Autodesk Inventor part; units mm, degrees
(part 3 of 4)
sketch "Sketch6" plane through (0, 0, 2) normal (0, 0, 1) x (1, 0, 0)
  line L0 (283.7872, -294.4284) -> (283.7872, -329.9768) projected
  line L1 (283.7872, -329.9768) -> (273.4247, -329.9768) projected
  line L2 (273.4247, -329.9768) -> (267.105, -323.7035) projected
  line L3 (267.105, -323.7035) -> (267.105, -286.25) projected
  line L4 (267.105, -286.25) -> (273.4247, -279.9768) projected
  line L5 (273.4247, -279.9768) -> (299.54, -279.9768) projected
  line L6 (299.54, -279.9768) -> (299.54, -294.4284) projected
  line L7 (299.54, -294.4284) -> (283.7872, -294.4284) projected
  line L8 (242.9879, -315.1998) -> (242.9879, -330.0232) projected
  line L9 (242.9879, -330.0232) -> (227.2351, -330.0232) projected
  line L10 (227.2351, -330.0232) -> (210.553, -313.3411) projected
  line L11 (210.553, -313.3411) -> (210.553, -279.9768) projected
  line L12 (210.553, -279.9768) -> (227.2351, -279.9768) projected
  line L13 (227.2351, -279.9768) -> (227.2351, -315.1998) projected
  line L14 (227.2351, -315.1998) -> (242.9879, -315.1998) projected
  line L15 (206.2779, -316.1756) -> (206.2779, -329.9768) projected
  line L16 (206.2779, -329.9768) -> (173.8429, -329.9768) projected
  line L17 (173.8429, -329.9768) -> (173.8429, -316.1756) projected
  line L18 (173.8429, -316.1756) -> (206.2779, -316.1756) projected
  line L19 (170.3113, -279.9768) -> (170.3113, -329.9768) projected
  line L20 (170.3113, -329.9768) -> (159.9954, -329.9768) projected
  line L21 (159.9954, -329.9768) -> (153.7221, -323.7035) projected
  line L22 (153.7221, -323.7035) -> (153.7221, -286.25) projected
  line L23 (153.7221, -286.25) -> (159.9954, -279.9768) projected
  line L24 (159.9954, -279.9768) -> (170.3113, -279.9768) projected
  line L25 (129.3262, -316.1292) -> (129.3262, -329.9303) projected
  line L26 (129.3262, -329.9303) -> (104.7444, -329.9303) projected
  line L27 (104.7444, -329.9303) -> (96.8913, -322.0771) projected
  line L28 (96.8913, -322.0771) -> (96.8913, -294.289) projected
  line L29 (96.8913, -294.289) -> (113.5734, -294.289) projected
  line L30 (113.5734, -294.289) -> (113.5734, -316.1292) projected
  line L31 (113.5734, -316.1292) -> (129.3262, -316.1292) projected
  line L32 (56.789, -329.9768) -> (46.6125, -329.9768) projected
  line L33 (46.6125, -329.9768) -> (40.3392, -323.7035) projected
  line L34 (40.3392, -323.7035) -> (40.3392, -279.9768) projected
  line L35 (40.3392, -279.9768) -> (56.789, -279.9768) projected
  line L36 (56.789, -279.9768) -> (56.789, -329.9768) projected
  line L37 (92.5697, -329.9768) -> (60.3206, -329.9768) projected
  line L38 (60.3206, -329.9768) -> (60.3206, -316.1756) projected
  line L39 (60.3206, -316.1756) -> (92.5697, -316.1756) projected
  line L40 (92.5697, -316.1756) -> (92.5697, -329.9768) projected
  line L41 (149.447, -294.289) -> (149.447, -329.9303) projected
  line L42 (149.447, -329.9303) -> (132.7649, -329.9303) projected
  line L43 (132.7649, -329.9303) -> (132.7649, -294.289) projected
  line L44 (132.7649, -294.289) -> (149.447, -294.289) projected
  line L45 (206.2779, -279.9768) -> (206.2779, -294.4284) projected
  line L46 (206.2779, -294.4284) -> (173.8429, -294.4284) projected
  line L47 (173.8429, -294.4284) -> (173.8429, -279.9768) projected
  line L48 (173.8429, -279.9768) -> (206.2779, -279.9768) projected
  line L49 (206.2779, -297.96) -> (206.2779, -308.973) projected
  line L50 (206.2779, -308.973) -> (173.8429, -308.973) projected
  line L51 (173.8429, -308.973) -> (173.8429, -297.96) projected
  line L52 (173.8429, -297.96) -> (206.2779, -297.96) projected
  line L53 (262.8299, -313.3411) -> (246.4266, -329.9768) projected
  line L54 (246.4266, -329.9768) -> (246.4266, -279.9768) projected
  line L55 (246.4266, -279.9768) -> (262.8299, -279.9768) projected
  line L56 (262.8299, -279.9768) -> (262.8299, -313.3411) projected
  line L57 (319.6608, -286.25) -> (319.6608, -323.7035) projected
  line L58 (319.6608, -323.7035) -> (313.3411, -329.9768) projected
  line L59 (313.3411, -329.9768) -> (287.1794, -329.9768) projected
  line L60 (287.1794, -329.9768) -> (287.1794, -316.1756) projected
  line L61 (287.1794, -316.1756) -> (302.9786, -316.1756) projected
  line L62 (302.9786, -316.1756) -> (302.9786, -279.9768) projected
  line L63 (302.9786, -279.9768) -> (313.3411, -279.9768) projected
  line L64 (313.3411, -279.9768) -> (319.6608, -286.25) projected
  line L65 (31.2247, -413) -> (28.338, -408) projected
  line L66 (28.338, -408) -> (31.2247, -403) projected
  line L67 (31.2247, -403) -> (36.9983, -403) projected
  line L68 (36.9983, -403) -> (39.885, -408) projected
  line L69 (39.885, -408) -> (36.9983, -413) projected
  line L70 (36.9983, -413) -> (31.2247, -413) projected
  line L71 (49.9886, -440.5) -> (52.8754, -445.5) projected
  line L72 (52.8754, -445.5) -> (49.9886, -450.5) projected
  line L73 (49.9886, -450.5) -> (44.2151, -450.5) projected
  line L74 (44.2151, -450.5) -> (41.3284, -445.5) projected
  line L75 (41.3284, -445.5) -> (44.2151, -440.5) projected
  line L76 (44.2151, -440.5) -> (49.9886, -440.5) projected
  line L77 (57.2247, -418) -> (62.9983, -418) projected
  line L78 (62.9983, -418) -> (65.885, -423) projected
  line L79 (65.885, -423) -> (62.9983, -428) projected
  line L80 (62.9983, -428) -> (57.2247, -428) projected
  line L81 (57.2247, -428) -> (54.338, -423) projected
  line L82 (54.338, -423) -> (57.2247, -418) projected
  line L83 (78.8754, -430.5) -> (75.9886, -435.5) projected
  line L84 (75.9886, -435.5) -> (70.2151, -435.5) projected
  line L85 (70.2151, -435.5) -> (67.3284, -430.5) projected
  line L86 (67.3284, -430.5) -> (70.2151, -425.5) projected
  line L87 (70.2151, -425.5) -> (75.9886, -425.5) projected
  line L88 (75.9886, -425.5) -> (78.8754, -430.5) projected
  line L89 (80.338, -438) -> (83.2247, -433) projected
  line L90 (83.2247, -433) -> (88.9983, -433) projected
  line L91 (88.9983, -433) -> (91.885, -438) projected
  line L92 (91.885, -438) -> (88.9983, -443) projected
  line L93 (88.9983, -443) -> (83.2247, -443) projected
  line L94 (83.2247, -443) -> (80.338, -438) projected
  line L95 (101.9886, -410.5) -> (104.8754, -415.5) projected
  line L96 (104.8754, -415.5) -> (101.9886, -420.5) projected
  line L97 (101.9886, -420.5) -> (96.2151, -420.5) projected
  line L98 (96.2151, -420.5) -> (93.3284, -415.5) projected
  line L99 (93.3284, -415.5) -> (96.2151, -410.5) projected
  line L100 (96.2151, -410.5) -> (101.9886, -410.5) projected
  line L101 (109.2247, -448) -> (114.9983, -448) projected
  line L102 (114.9983, -448) -> (117.885, -453) projected
  line L103 (117.885, -453) -> (114.9983, -458) projected
  line L104 (114.9983, -458) -> (109.2247, -458) projected
  line L105 (109.2247, -458) -> (106.338, -453) projected
  line L106 (106.338, -453) -> (109.2247, -448) projected
  line L107 (135.2247, -413) -> (132.338, -408) projected
  line L108 (132.338, -408) -> (135.2247, -403) projected
  line L109 (135.2247, -403) -> (140.9983, -403) projected
  line L110 (140.9983, -403) -> (143.885, -408) projected
  line L111 (143.885, -408) -> (140.9983, -413) projected
  line L112 (140.9983, -413) -> (135.2247, -413) projected
  line L113 (153.9886, -440.5) -> (156.8754, -445.5) projected
  line L114 (156.8754, -445.5) -> (153.9886, -450.5) projected
  line L115 (153.9886, -450.5) -> (148.2151, -450.5) projected
  line L116 (148.2151, -450.5) -> (145.3284, -445.5) projected
  line L117 (145.3284, -445.5) -> (148.2151, -440.5) projected
  line L118 (148.2151, -440.5) -> (153.9886, -440.5) projected
  line L119 (153.9886, -410.5) -> (156.8754, -415.5) projected
  line L120 (156.8754, -415.5) -> (153.9886, -420.5) projected
  line L121 (153.9886, -420.5) -> (148.2151, -420.5) projected
  line L122 (148.2151, -420.5) -> (145.3284, -415.5) projected
  line L123 (145.3284, -415.5) -> (148.2151, -410.5) projected
  line L124 (148.2151, -410.5) -> (153.9886, -410.5) projected
  line L125 (182.8754, -430.5) -> (179.9886, -435.5) projected
  line L126 (179.9886, -435.5) -> (174.2151, -435.5) projected
  line L127 (174.2151, -435.5) -> (171.3284, -430.5) projected
  line L128 (171.3284, -430.5) -> (174.2151, -425.5) projected
  line L129 (174.2151, -425.5) -> (179.9886, -425.5) projected
  line L130 (179.9886, -425.5) -> (182.8754, -430.5) projected
  line L131 (184.338, -438) -> (187.2247, -433) projected
  line L132 (187.2247, -433) -> (192.9983, -433) projected
  line L133 (192.9983, -433) -> (195.885, -438) projected
  line L134 (195.885, -438) -> (192.9983, -443) projected
  line L135 (192.9983, -443) -> (187.2247, -443) projected
  line L136 (187.2247, -443) -> (184.338, -438) projected
  line L137 (205.9886, -410.5) -> (208.8754, -415.5) projected
  line L138 (208.8754, -415.5) -> (205.9886, -420.5) projected
  line L139 (205.9886, -420.5) -> (200.2151, -420.5) projected
  line L140 (200.2151, -420.5) -> (197.3284, -415.5) projected
  line L141 (197.3284, -415.5) -> (200.2151, -410.5) projected
  line L142 (200.2151, -410.5) -> (205.9886, -410.5) projected
  line L143 (213.2247, -448) -> (218.9983, -448) projected
  line L144 (218.9983, -448) -> (221.885, -453) projected
  line L145 (221.885, -453) -> (218.9983, -458) projected
  line L146 (218.9983, -458) -> (213.2247, -458) projected
  line L147 (213.2247, -458) -> (210.338, -453) projected
  line L148 (210.338, -453) -> (213.2247, -448) projected
  line L149 (239.2247, -413) -> (236.338, -408) projected
  line L150 (236.338, -408) -> (239.2247, -403) projected
  line L151 (239.2247, -403) -> (244.9983, -403) projected
  line L152 (244.9983, -403) -> (247.885, -408) projected
  line L153 (247.885, -408) -> (244.9983, -413) projected
  line L154 (244.9983, -413) -> (239.2247, -413) projected
  line L155 (257.9886, -440.5) -> (260.8754, -445.5) projected
  line L156 (260.8754, -445.5) -> (257.9886, -450.5) projected
  line L157 (257.9886, -450.5) -> (252.2151, -450.5) projected
  line L158 (252.2151, -450.5) -> (249.3284, -445.5) projected
  line L159 (249.3284, -445.5) -> (252.2151, -440.5) projected
  line L160 (252.2151, -440.5) -> (257.9886, -440.5) projected
  line L161 (265.2247, -418) -> (270.9983, -418) projected
  line L162 (270.9983, -418) -> (273.885, -423) projected
  line L163 (273.885, -423) -> (270.9983, -428) projected
  line L164 (270.9983, -428) -> (265.2247, -428) projected
  line L165 (265.2247, -428) -> (262.338, -423) projected
  line L166 (262.338, -423) -> (265.2247, -418) projected
  line L167 (291.2247, -448) -> (296.9983, -448) projected
  line L168 (296.9983, -448) -> (299.885, -453) projected
  line L169 (299.885, -453) -> (296.9983, -458) projected
  line L170 (296.9983, -458) -> (291.2247, -458) projected
  line L171 (291.2247, -458) -> (288.338, -453) projected
  line L172 (288.338, -453) -> (291.2247, -448) projected
  line L173 (343.2247, -448) -> (348.9983, -448) projected
  line L174 (348.9983, -448) -> (351.885, -453) projected
  line L175 (351.885, -453) -> (348.9983, -458) projected
  line L176 (348.9983, -458) -> (343.2247, -458) projected
  line L177 (343.2247, -458) -> (340.338, -453) projected
  line L178 (340.338, -453) -> (343.2247, -448) projected
  line L179 (335.9886, -410.5) -> (338.8754, -415.5) projected
  line L180 (338.8754, -415.5) -> (335.9886, -420.5) projected
  line L181 (335.9886, -420.5) -> (330.2151, -420.5) projected
  line L182 (330.2151, -420.5) -> (327.3284, -415.5) projected
  line L183 (327.3284, -415.5) -> (330.2151, -410.5) projected
  line L184 (330.2151, -410.5) -> (335.9886, -410.5) projected
  line L185 (286.8754, -430.5) -> (283.9886, -435.5) projected
  line L186 (283.9886, -435.5) -> (278.2151, -435.5) projected
  line L187 (278.2151, -435.5) -> (275.3284, -430.5) projected
  line L188 (275.3284, -430.5) -> (278.2151, -425.5) projected
  line L189 (278.2151, -425.5) -> (283.9886, -425.5) projected
  line L190 (283.9886, -425.5) -> (286.8754, -430.5) projected
  line L191 (309.9886, -410.5) -> (312.8754, -415.5) projected
  line L192 (312.8754, -415.5) -> (309.9886, -420.5) projected
  line L193 (309.9886, -420.5) -> (304.2151, -420.5) projected
  line L194 (304.2151, -420.5) -> (301.3284, -415.5) projected
  line L195 (301.3284, -415.5) -> (304.2151, -410.5) projected
  line L196 (304.2151, -410.5) -> (309.9886, -410.5) projected
  line L197 (5.2247, -433) -> (10.9983, -433) projected
  line L198 (10.9983, -433) -> (13.885, -438) projected
  line L199 (13.885, -438) -> (10.9983, -443) projected
  line L200 (10.9983, -443) -> (5.2247, -443) projected
  line L201 (5.2247, -443) -> (2.338, -438) projected
  line L202 (2.338, -438) -> (5.2247, -433) projected
  line L203 (23.9886, -440.5) -> (26.8754, -445.5) projected
  line L204 (26.8754, -445.5) -> (23.9886, -450.5) projected
  line L205 (23.9886, -450.5) -> (18.2151, -450.5) projected
  line L206 (18.2151, -450.5) -> (15.3284, -445.5) projected
  line L207 (15.3284, -445.5) -> (18.2151, -440.5) projected
  line L208 (18.2151, -440.5) -> (23.9886, -440.5) projected
  line L209 (10.9983, -428) -> (5.2247, -428) projected
  line L210 (5.2247, -428) -> (2.338, -423) projected
  line L211 (2.338, -423) -> (5.2247, -418) projected
  line L212 (5.2247, -418) -> (10.9983, -418) projected
  line L213 (10.9983, -418) -> (13.885, -423) projected
  line L214 (13.885, -423) -> (10.9983, -428) projected
  line L215 (317.2247, -418) -> (322.9983, -418) projected
  line L216 (322.9983, -418) -> (325.885, -423) projected
  line L217 (325.885, -423) -> (322.9983, -428) projected
  line L218 (322.9983, -428) -> (317.2247, -428) projected
  line L219 (317.2247, -428) -> (314.338, -423) projected
  line L220 (314.338, -423) -> (317.2247, -418) projected
  line L221 (291.2247, -418) -> (296.9983, -418) projected
  line L222 (296.9983, -418) -> (299.885, -423) projected
  line L223 (299.885, -423) -> (296.9983, -428) projected
  line L224 (296.9983, -428) -> (291.2247, -428) projected
  line L225 (291.2247, -428) -> (288.338, -423) projected
  line L226 (288.338, -423) -> (291.2247, -418) projected
  line L227 (317.2247, -413) -> (314.338, -408) projected
  line L228 (314.338, -408) -> (317.2247, -403) projected
  line L229 (317.2247, -403) -> (322.9983, -403) projected
  line L230 (322.9983, -403) -> (325.885, -408) projected
  line L231 (325.885, -408) -> (322.9983, -413) projected
  line L232 (322.9983, -413) -> (317.2247, -413) projected
  line L233 (340.338, -438) -> (343.2247, -433) projected
  line L234 (343.2247, -433) -> (348.9983, -433) projected
  line L235 (348.9983, -433) -> (351.885, -438) projected
  line L236 (351.885, -438) -> (348.9983, -443) projected
  line L237 (348.9983, -443) -> (343.2247, -443) projected
  line L238 (343.2247, -443) -> (340.338, -438) projected
  line L239 (309.9886, -440.5) -> (312.8754, -445.5) projected
  line L240 (312.8754, -445.5) -> (309.9886, -450.5) projected
  line L241 (309.9886, -450.5) -> (304.2151, -450.5) projected
  line L242 (304.2151, -450.5) -> (301.3284, -445.5) projected
  line L243 (301.3284, -445.5) -> (304.2151, -440.5) projected
  line L244 (304.2151, -440.5) -> (309.9886, -440.5) projected
  line L245 (262.338, -438) -> (265.2247, -433) projected
  line L246 (265.2247, -433) -> (270.9983, -433) projected
  line L247 (270.9983, -433) -> (273.885, -438) projected
  line L248 (273.885, -438) -> (270.9983, -443) projected
  line L249 (270.9983, -443) -> (265.2247, -443) projected
  line L250 (265.2247, -443) -> (262.338, -438) projected
  line L251 (260.8754, -430.5) -> (257.9886, -435.5) projected
  line L252 (257.9886, -435.5) -> (252.2151, -435.5) projected
  line L253 (252.2151, -435.5) -> (249.3284, -430.5) projected
  line L254 (249.3284, -430.5) -> (252.2151, -425.5) projected
  line L255 (252.2151, -425.5) -> (257.9886, -425.5) projected
  line L256 (257.9886, -425.5) -> (260.8754, -430.5) projected
  line L257 (239.2247, -418) -> (244.9983, -418) projected
  line L258 (244.9983, -418) -> (247.885, -423) projected
  line L259 (247.885, -423) -> (244.9983, -428) projected
  line L260 (244.9983, -428) -> (239.2247, -428) projected
  line L261 (239.2247, -428) -> (236.338, -423) projected
  line L262 (236.338, -423) -> (239.2247, -418) projected
  line L263 (231.9886, -440.5) -> (234.8754, -445.5) projected
  line L264 (234.8754, -445.5) -> (231.9886, -450.5) projected
  line L265 (231.9886, -450.5) -> (226.2151, -450.5) projected
  line L266 (226.2151, -450.5) -> (223.3284, -445.5) projected
  line L267 (223.3284, -445.5) -> (226.2151, -440.5) projected
  line L268 (226.2151, -440.5) -> (231.9886, -440.5) projected
  line L269 (213.2247, -413) -> (210.338, -408) projected
  line L270 (210.338, -408) -> (213.2247, -403) projected
  line L271 (213.2247, -403) -> (218.9983, -403) projected
  line L272 (218.9983, -403) -> (221.885, -408) projected
  line L273 (221.885, -408) -> (218.9983, -413) projected
  line L274 (218.9983, -413) -> (213.2247, -413) projected
  line L275 (187.2247, -448) -> (192.9983, -448) projected
  line L276 (192.9983, -448) -> (195.885, -453) projected
  line L277 (195.885, -453) -> (192.9983, -458) projected
  line L278 (192.9983, -458) -> (187.2247, -458) projected
  line L279 (187.2247, -458) -> (184.338, -453) projected
  line L280 (184.338, -453) -> (187.2247, -448) projected
  line L281 (179.9886, -410.5) -> (182.8754, -415.5) projected
  line L282 (182.8754, -415.5) -> (179.9886, -420.5) projected
  line L283 (179.9886, -420.5) -> (174.2151, -420.5) projected
  line L284 (174.2151, -420.5) -> (171.3284, -415.5) projected
  line L285 (171.3284, -415.5) -> (174.2151, -410.5) projected
  line L286 (174.2151, -410.5) -> (179.9886, -410.5) projected
  line L287 (161.2247, -413) -> (158.338, -408) projected
  line L288 (158.338, -408) -> (161.2247, -403) projected
  line L289 (161.2247, -403) -> (166.9983, -403) projected
  line L290 (166.9983, -403) -> (169.885, -408) projected
  line L291 (169.885, -408) -> (166.9983, -413) projected
  line L292 (166.9983, -413) -> (161.2247, -413) projected
  line L293 (161.2247, -448) -> (166.9983, -448) projected
  line L294 (166.9983, -448) -> (169.885, -453) projected
  line L295 (169.885, -453) -> (166.9983, -458) projected
  line L296 (166.9983, -458) -> (161.2247, -458) projected
  line L297 (161.2247, -458) -> (158.338, -453) projected
  line L298 (158.338, -453) -> (161.2247, -448) projected
  line L299 (135.2247, -418) -> (140.9983, -418) projected
  line L300 (140.9983, -418) -> (143.885, -423) projected
  line L301 (143.885, -423) -> (140.9983, -428) projected
  line L302 (140.9983, -428) -> (135.2247, -428) projected
  line L303 (135.2247, -428) -> (132.338, -423) projected
  line L304 (132.338, -423) -> (135.2247, -418) projected
  line L305 (127.9886, -440.5) -> (130.8754, -445.5) projected
  line L306 (130.8754, -445.5) -> (127.9886, -450.5) projected
  line L307 (127.9886, -450.5) -> (122.2151, -450.5) projected
  line L308 (122.2151, -450.5) -> (119.3284, -445.5) projected
  line L309 (119.3284, -445.5) -> (122.2151, -440.5) projected
  line L310 (122.2151, -440.5) -> (127.9886, -440.5) projected
  line L311 (109.2247, -413) -> (106.338, -408) projected
  line L312 (106.338, -408) -> (109.2247, -403) projected
  line L313 (109.2247, -403) -> (114.9983, -403) projected
  line L314 (114.9983, -403) -> (117.885, -408) projected
  line L315 (117.885, -408) -> (114.9983, -413) projected
  line L316 (114.9983, -413) -> (109.2247, -413) projected
  line L317 (83.2247, -448) -> (88.9983, -448) projected
  line L318 (88.9983, -448) -> (91.885, -453) projected
  line L319 (91.885, -453) -> (88.9983, -458) projected
  line L320 (88.9983, -458) -> (83.2247, -458) projected
  line L321 (83.2247, -458) -> (80.338, -453) projected
  line L322 (80.338, -453) -> (83.2247, -448) projected
  line L323 (75.9886, -410.5) -> (78.8754, -415.5) projected
  line L324 (78.8754, -415.5) -> (75.9886, -420.5) projected
  line L325 (75.9886, -420.5) -> (70.2151, -420.5) projected
  line L326 (70.2151, -420.5) -> (67.3284, -415.5) projected
  line L327 (67.3284, -415.5) -> (70.2151, -410.5) projected
  line L328 (70.2151, -410.5) -> (75.9886, -410.5) projected
  line L329 (54.338, -438) -> (57.2247, -433) projected
  line L330 (57.2247, -433) -> (62.9983, -433) projected
  line L331 (62.9983, -433) -> (65.885, -438) projected
  line L332 (65.885, -438) -> (62.9983, -443) projected
  line L333 (62.9983, -443) -> (57.2247, -443) projected
  line L334 (57.2247, -443) -> (54.338, -438) projected
  line L335 (52.8754, -430.5) -> (49.9886, -435.5) projected
  line L336 (49.9886, -435.5) -> (44.2151, -435.5) projected
  line L337 (44.2151, -435.5) -> (41.3284, -430.5) projected
  line L338 (41.3284, -430.5) -> (44.2151, -425.5) projected
  line L339 (44.2151, -425.5) -> (49.9886, -425.5) projected
  line L340 (49.9886, -425.5) -> (52.8754, -430.5) projected
  line L341 (31.2247, -418) -> (36.9983, -418) projected
  line L342 (36.9983, -418) -> (39.885, -423) projected
  line L343 (39.885, -423) -> (36.9983, -428) projected
  line L344 (36.9983, -428) -> (31.2247, -428) projected
  line L345 (31.2247, -428) -> (28.338, -423) projected
  line L346 (28.338, -423) -> (31.2247, -418) projected
  line L347 (23.9886, -420.5) -> (18.2151, -420.5) projected
  line L348 (18.2151, -420.5) -> (15.3284, -415.5) projected
  line L349 (15.3284, -415.5) -> (18.2151, -410.5) projected
  line L350 (18.2151, -410.5) -> (23.9886, -410.5) projected
  line L351 (23.9886, -410.5) -> (26.8754, -415.5) projected
  line L352 (26.8754, -415.5) -> (23.9886, -420.5) projected
  line L353 (31.2247, -448) -> (36.9983, -448) projected
  line L354 (36.9983, -448) -> (39.885, -453) projected
  line L355 (39.885, -453) -> (36.9983, -458) projected
  line L356 (36.9983, -458) -> (31.2247, -458) projected
  line L357 (31.2247, -458) -> (28.338, -453) projected
  line L358 (28.338, -453) -> (31.2247, -448) projected
  line L359 (57.2247, -413) -> (54.338, -408) projected
  line L360 (54.338, -408) -> (57.2247, -403) projected
  line L361 (57.2247, -403) -> (62.9983, -403) projected
  line L362 (62.9983, -403) -> (65.885, -408) projected
  line L363 (65.885, -408) -> (62.9983, -413) projected
  line L364 (62.9983, -413) -> (57.2247, -413) projected
  line L365 (75.9886, -440.5) -> (78.8754, -445.5) projected
  line L366 (78.8754, -445.5) -> (75.9886, -450.5) projected
  line L367 (75.9886, -450.5) -> (70.2151, -450.5) projected
  line L368 (70.2151, -450.5) -> (67.3284, -445.5) projected
  line L369 (67.3284, -445.5) -> (70.2151, -440.5) projected
  line L370 (70.2151, -440.5) -> (75.9886, -440.5) projected
  line L371 (83.2247, -418) -> (88.9983, -418) projected
  line L372 (88.9983, -418) -> (91.885, -423) projected
  line L373 (91.885, -423) -> (88.9983, -428) projected
  line L374 (88.9983, -428) -> (83.2247, -428) projected
  line L375 (83.2247, -428) -> (80.338, -423) projected
  line L376 (80.338, -423) -> (83.2247, -418) projected
  line L377 (104.8754, -430.5) -> (101.9886, -435.5) projected
  line L378 (101.9886, -435.5) -> (96.2151, -435.5) projected
  line L379 (96.2151, -435.5) -> (93.3284, -430.5) projected
  line L380 (93.3284, -430.5) -> (96.2151, -425.5) projected
  line L381 (96.2151, -425.5) -> (101.9886, -425.5) projected
  line L382 (101.9886, -425.5) -> (104.8754, -430.5) projected
  line L383 (106.338, -438) -> (109.2247, -433) projected
  line L384 (109.2247, -433) -> (114.9983, -433) projected
  line L385 (114.9983, -433) -> (117.885, -438) projected
  line L386 (117.885, -438) -> (114.9983, -443) projected
  line L387 (114.9983, -443) -> (109.2247, -443) projected
  line L388 (109.2247, -443) -> (106.338, -438) projected
  line L389 (127.9886, -410.5) -> (130.8754, -415.5) projected
  line L390 (130.8754, -415.5) -> (127.9886, -420.5) projected
  line L391 (127.9886, -420.5) -> (122.2151, -420.5) projected
  line L392 (122.2151, -420.5) -> (119.3284, -415.5) projected
  line L393 (119.3284, -415.5) -> (122.2151, -410.5) projected
  line L394 (122.2151, -410.5) -> (127.9886, -410.5) projected
  line L395 (135.2247, -448) -> (140.9983, -448) projected
  line L396 (140.9983, -448) -> (143.885, -453) projected
  line L397 (143.885, -453) -> (140.9983, -458) projected
  line L398 (140.9983, -458) -> (135.2247, -458) projected
  line L399 (135.2247, -458) -> (132.338, -453) projected
  line L400 (132.338, -453) -> (135.2247, -448) projected
  line L401 (156.8754, -430.5) -> (153.9886, -435.5) projected
  line L402 (153.9886, -435.5) -> (148.2151, -435.5) projected
  line L403 (148.2151, -435.5) -> (145.3284, -430.5) projected
  line L404 (145.3284, -430.5) -> (148.2151, -425.5) projected
  line L405 (148.2151, -425.5) -> (153.9886, -425.5) projected
  line L406 (153.9886, -425.5) -> (156.8754, -430.5) projected
  line L407 (179.9886, -440.5) -> (182.8754, -445.5) projected
  line L408 (182.8754, -445.5) -> (179.9886, -450.5) projected
  line L409 (179.9886, -450.5) -> (174.2151, -450.5) projected
  line L410 (174.2151, -450.5) -> (171.3284, -445.5) projected
  line L411 (171.3284, -445.5) -> (174.2151, -440.5) projected
  line L412 (174.2151, -440.5) -> (179.9886, -440.5) projected
  line L413 (187.2247, -418) -> (192.9983, -418) projected
  line L414 (192.9983, -418) -> (195.885, -423) projected
  line L415 (195.885, -423) -> (192.9983, -428) projected
  line L416 (192.9983, -428) -> (187.2247, -428) projected
  line L417 (187.2247, -428) -> (184.338, -423) projected
  line L418 (184.338, -423) -> (187.2247, -418) projected
  line L419 (208.8754, -430.5) -> (205.9886, -435.5) projected
  line L420 (205.9886, -435.5) -> (200.2151, -435.5) projected
  line L421 (200.2151, -435.5) -> (197.3284, -430.5) projected
  line L422 (197.3284, -430.5) -> (200.2151, -425.5) projected
  line L423 (200.2151, -425.5) -> (205.9886, -425.5) projected
  line L424 (205.9886, -425.5) -> (208.8754, -430.5) projected
  line L425 (210.338, -438) -> (213.2247, -433) projected
  line L426 (213.2247, -433) -> (218.9983, -433) projected
  line L427 (218.9983, -433) -> (221.885, -438) projected
  line L428 (221.885, -438) -> (218.9983, -443) projected
  line L429 (218.9983, -443) -> (213.2247, -443) projected
  line L430 (213.2247, -443) -> (210.338, -438) projected
  line L431 (231.9886, -410.5) -> (234.8754, -415.5) projected
  line L432 (234.8754, -415.5) -> (231.9886, -420.5) projected
  line L433 (231.9886, -420.5) -> (226.2151, -420.5) projected
  line L434 (226.2151, -420.5) -> (223.3284, -415.5) projected
  line L435 (223.3284, -415.5) -> (226.2151, -410.5) projected
  line L436 (226.2151, -410.5) -> (231.9886, -410.5) projected
  line L437 (239.2247, -448) -> (244.9983, -448) projected
  line L438 (244.9983, -448) -> (247.885, -453) projected
  line L439 (247.885, -453) -> (244.9983, -458) projected
  line L440 (244.9983, -458) -> (239.2247, -458) projected
  line L441 (239.2247, -458) -> (236.338, -453) projected
  line L442 (236.338, -453) -> (239.2247, -448) projected
  line L443 (265.2247, -413) -> (262.338, -408) projected
  line L444 (262.338, -408) -> (265.2247, -403) projected
  line L445 (265.2247, -403) -> (270.9983, -403) projected
  line L446 (270.9983, -403) -> (273.885, -408) projected
  line L447 (273.885, -408) -> (270.9983, -413) projected
  line L448 (270.9983, -413) -> (265.2247, -413) projected
  line L449 (283.9886, -440.5) -> (286.8754, -445.5) projected
  line L450 (286.8754, -445.5) -> (283.9886, -450.5) projected
  line L451 (283.9886, -450.5) -> (278.2151, -450.5) projected
  line L452 (278.2151, -450.5) -> (275.3284, -445.5) projected
  line L453 (275.3284, -445.5) -> (278.2151, -440.5) projected
  line L454 (278.2151, -440.5) -> (283.9886, -440.5) projected
  line L455 (335.9886, -440.5) -> (338.8754, -445.5) projected
  line L456 (338.8754, -445.5) -> (335.9886, -450.5) projected
  line L457 (335.9886, -450.5) -> (330.2151, -450.5) projected
  line L458 (330.2151, -450.5) -> (327.3284, -445.5) projected
  line L459 (327.3284, -445.5) -> (330.2151, -440.5) projected
  line L460 (330.2151, -440.5) -> (335.9886, -440.5) projected
  line L461 (343.2247, -413) -> (340.338, -408) projected
  line L462 (340.338, -408) -> (343.2247, -403) projected
  line L463 (343.2247, -403) -> (348.9983, -403) projected
  line L464 (348.9983, -403) -> (351.885, -408) projected
  line L465 (351.885, -408) -> (348.9983, -413) projected
  line L466 (348.9983, -413) -> (343.2247, -413) projected
  line L467 (283.9886, -410.5) -> (286.8754, -415.5) projected
  line L468 (286.8754, -415.5) -> (283.9886, -420.5) projected
  line L469 (283.9886, -420.5) -> (278.2151, -420.5) projected
  line L470 (278.2151, -420.5) -> (275.3284, -415.5) projected
  line L471 (275.3284, -415.5) -> (278.2151, -410.5) projected
  line L472 (278.2151, -410.5) -> (283.9886, -410.5) projected
  line L473 (312.8754, -430.5) -> (309.9886, -435.5) projected
  line L474 (309.9886, -435.5) -> (304.2151, -435.5) projected
  line L475 (304.2151, -435.5) -> (301.3284, -430.5) projected
  line L476 (301.3284, -430.5) -> (304.2151, -425.5) projected
  line L477 (304.2151, -425.5) -> (309.9886, -425.5) projected
  line L478 (309.9886, -425.5) -> (312.8754, -430.5) projected
  line L479 (338.8754, -430.5) -> (335.9886, -435.5) projected
  line L480 (335.9886, -435.5) -> (330.2151, -435.5) projected
  line L481 (330.2151, -435.5) -> (327.3284, -430.5) projected
  line L482 (327.3284, -430.5) -> (330.2151, -425.5) projected
  line L483 (330.2151, -425.5) -> (335.9886, -425.5) projected
  line L484 (335.9886, -425.5) -> (338.8754, -430.5) projected
  line L485 (23.9886, -435.5) -> (18.2151, -435.5) projected
  line L486 (18.2151, -435.5) -> (15.3284, -430.5) projected
  line L487 (15.3284, -430.5) -> (18.2151, -425.5) projected
  line L488 (18.2151, -425.5) -> (23.9886, -425.5) projected
  line L489 (23.9886, -425.5) -> (26.8754, -430.5) projected
  line L490 (26.8754, -430.5) -> (23.9886, -435.5) projected
  line L491 (5.2247, -448) -> (10.9983, -448) projected
  line L492 (10.9983, -448) -> (13.885, -453) projected
  line L493 (13.885, -453) -> (10.9983, -458) projected
  line L494 (10.9983, -458) -> (5.2247, -458) projected
  line L495 (5.2247, -458) -> (2.338, -453) projected
  line L496 (2.338, -453) -> (5.2247, -448) projected
  line L497 (314.338, -438) -> (317.2247, -433) projected
  line L498 (317.2247, -433) -> (322.9983, -433) projected
  line L499 (322.9983, -433) -> (325.885, -438) projected
  line L500 (325.885, -438) -> (322.9983, -443) projected
  line L501 (322.9983, -443) -> (317.2247, -443) projected
  line L502 (317.2247, -443) -> (314.338, -438) projected
  line L503 (288.338, -438) -> (291.2247, -433) projected
  line L504 (291.2247, -433) -> (296.9983, -433) projected
  line L505 (296.9983, -433) -> (299.885, -438) projected
  line L506 (299.885, -438) -> (296.9983, -443) projected
  line L507 (296.9983, -443) -> (291.2247, -443) projected
  line L508 (291.2247, -443) -> (288.338, -438) projected
  line L509 (291.2247, -413) -> (288.338, -408) projected
  line L510 (288.338, -408) -> (291.2247, -403) projected
  line L511 (291.2247, -403) -> (296.9983, -403) projected
  line L512 (296.9983, -403) -> (299.885, -408) projected
  line L513 (299.885, -408) -> (296.9983, -413) projected
  line L514 (296.9983, -413) -> (291.2247, -413) projected
  line L515 (343.2247, -418) -> (348.9983, -418) projected
  line L516 (348.9983, -418) -> (351.885, -423) projected
  line L517 (351.885, -423) -> (348.9983, -428) projected
  line L518 (348.9983, -428) -> (343.2247, -428) projected
  line L519 (343.2247, -428) -> (340.338, -423) projected
  line L520 (340.338, -423) -> (343.2247, -418) projected
  line L521 (317.2247, -448) -> (322.9983, -448) projected
  line L522 (322.9983, -448) -> (325.885, -453) projected
  line L523 (325.885, -453) -> (322.9983, -458) projected
  line L524 (322.9983, -458) -> (317.2247, -458) projected
  line L525 (317.2247, -458) -> (314.338, -453) projected
  line L526 (314.338, -453) -> (317.2247, -448) projected
  line L527 (265.2247, -448) -> (270.9983, -448) projected
  line L528 (270.9983, -448) -> (273.885, -453) projected
  line L529 (273.885, -453) -> (270.9983, -458) projected
  line L530 (270.9983, -458) -> (265.2247, -458) projected
  line L531 (265.2247, -458) -> (262.338, -453) projected
  line L532 (262.338, -453) -> (265.2247, -448) projected
  line L533 (257.9886, -410.5) -> (260.8754, -415.5) projected
  line L534 (260.8754, -415.5) -> (257.9886, -420.5) projected
  line L535 (257.9886, -420.5) -> (252.2151, -420.5) projected
  line L536 (252.2151, -420.5) -> (249.3284, -415.5) projected
  line L537 (249.3284, -415.5) -> (252.2151, -410.5) projected
  line L538 (252.2151, -410.5) -> (257.9886, -410.5) projected
  line L539 (236.338, -438) -> (239.2247, -433) projected
  line L540 (239.2247, -433) -> (244.9983, -433) projected
  line L541 (244.9983, -433) -> (247.885, -438) projected
  line L542 (247.885, -438) -> (244.9983, -443) projected
  line L543 (244.9983, -443) -> (239.2247, -443) projected
  line L544 (239.2247, -443) -> (236.338, -438) projected
  line L545 (234.8754, -430.5) -> (231.9886, -435.5) projected
  line L546 (231.9886, -435.5) -> (226.2151, -435.5) projected
  line L547 (226.2151, -435.5) -> (223.3284, -430.5) projected
  line L548 (223.3284, -430.5) -> (226.2151, -425.5) projected
  line L549 (226.2151, -425.5) -> (231.9886, -425.5) projected
  line L550 (231.9886, -425.5) -> (234.8754, -430.5) projected
  line L551 (213.2247, -418) -> (218.9983, -418) projected
  line L552 (218.9983, -418) -> (221.885, -423) projected
  line L553 (221.885, -423) -> (218.9983, -428) projected
  line L554 (218.9983, -428) -> (213.2247, -428) projected
  line L555 (213.2247, -428) -> (210.338, -423) projected
  line L556 (210.338, -423) -> (213.2247, -418) projected
  line L557 (205.9886, -440.5) -> (208.8754, -445.5) projected
  line L558 (208.8754, -445.5) -> (205.9886, -450.5) projected
  line L559 (205.9886, -450.5) -> (200.2151, -450.5) projected
  line L560 (200.2151, -450.5) -> (197.3284, -445.5) projected
  line L561 (197.3284, -445.5) -> (200.2151, -440.5) projected
  line L562 (200.2151, -440.5) -> (205.9886, -440.5) projected
  line L563 (187.2247, -413) -> (184.338, -408) projected
  line L564 (184.338, -408) -> (187.2247, -403) projected
  line L565 (187.2247, -403) -> (192.9983, -403) projected
  line L566 (192.9983, -403) -> (195.885, -408) projected
  line L567 (195.885, -408) -> (192.9983, -413) projected
  line L568 (192.9983, -413) -> (187.2247, -413) projected
  line L569 (161.2247, -418) -> (166.9983, -418) projected
  line L570 (166.9983, -418) -> (169.885, -423) projected
  line L571 (169.885, -423) -> (166.9983, -428) projected
  line L572 (166.9983, -428) -> (161.2247, -428) projected
  line L573 (161.2247, -428) -> (158.338, -423) projected
  line L574 (158.338, -423) -> (161.2247, -418) projected
  line L575 (158.338, -438) -> (161.2247, -433) projected
  line L576 (161.2247, -433) -> (166.9983, -433) projected
  line L577 (166.9983, -433) -> (169.885, -438) projected
  line L578 (169.885, -438) -> (166.9983, -443) projected
  line L579 (166.9983, -443) -> (161.2247, -443) projected
  line L580 (161.2247, -443) -> (158.338, -438) projected
  line L581 (132.338, -438) -> (135.2247, -433) projected
  line L582 (135.2247, -433) -> (140.9983, -433) projected
  line L583 (140.9983, -433) -> (143.885, -438) projected
  line L584 (143.885, -438) -> (140.9983, -443) projected
  line L585 (140.9983, -443) -> (135.2247, -443) projected
  line L586 (135.2247, -443) -> (132.338, -438) projected
  line L587 (130.8754, -430.5) -> (127.9886, -435.5) projected
  line L588 (127.9886, -435.5) -> (122.2151, -435.5) projected
  line L589 (122.2151, -435.5) -> (119.3284, -430.5) projected
  line L590 (119.3284, -430.5) -> (122.2151, -425.5) projected
  line L591 (122.2151, -425.5) -> (127.9886, -425.5) projected
  line L592 (127.9886, -425.5) -> (130.8754, -430.5) projected
  line L593 (109.2247, -418) -> (114.9983, -418) projected
  line L594 (114.9983, -418) -> (117.885, -423) projected
  line L595 (117.885, -423) -> (114.9983, -428) projected
  line L596 (114.9983, -428) -> (109.2247, -428) projected
  line L597 (109.2247, -428) -> (106.338, -423) projected
  line L598 (106.338, -423) -> (109.2247, -418) projected
  line L599 (101.9886, -440.5) -> (104.8754, -445.5) projected
  line L600 (104.8754, -445.5) -> (101.9886, -450.5) projected
  line L601 (101.9886, -450.5) -> (96.2151, -450.5) projected
  line L602 (96.2151, -450.5) -> (93.3284, -445.5) projected
  line L603 (93.3284, -445.5) -> (96.2151, -440.5) projected
  line L604 (96.2151, -440.5) -> (101.9886, -440.5) projected
  line L605 (83.2247, -413) -> (80.338, -408) projected
  line L606 (80.338, -408) -> (83.2247, -403) projected
  line L607 (83.2247, -403) -> (88.9983, -403) projected
  line L608 (88.9983, -403) -> (91.885, -408) projected
  line L609 (91.885, -408) -> (88.9983, -413) projected
  line L610 (88.9983, -413) -> (83.2247, -413) projected
  line L611 (57.2247, -448) -> (62.9983, -448) projected
  line L612 (62.9983, -448) -> (65.885, -453) projected
  line L613 (65.885, -453) -> (62.9983, -458) projected
  line L614 (62.9983, -458) -> (57.2247, -458) projected
  line L615 (57.2247, -458) -> (54.338, -453) projected
  line L616 (54.338, -453) -> (57.2247, -448) projected
  line L617 (49.9886, -410.5) -> (52.8754, -415.5) projected
  line L618 (52.8754, -415.5) -> (49.9886, -420.5) projected
  line L619 (49.9886, -420.5) -> (44.2151, -420.5) projected
  line L620 (44.2151, -420.5) -> (41.3284, -415.5) projected
  line L621 (41.3284, -415.5) -> (44.2151, -410.5) projected
  line L622 (44.2151, -410.5) -> (49.9886, -410.5) projected
  line L623 (28.338, -438) -> (31.2247, -433) projected
  line L624 (31.2247, -433) -> (36.9983, -433) projected
  line L625 (36.9983, -433) -> (39.885, -438) projected
  line L626 (39.885, -438) -> (36.9983, -443) projected
  line L627 (36.9983, -443) -> (31.2247, -443) projected
  line L628 (31.2247, -443) -> (28.338, -438) projected
  line L629 (10.9983, -413) -> (5.2247, -413) projected
  line L630 (5.2247, -413) -> (2.338, -408) projected
  line L631 (2.338, -408) -> (5.2247, -403) projected
  line L632 (5.2247, -403) -> (10.9983, -403) projected
  line L633 (10.9983, -403) -> (13.885, -408) projected
  line L634 (13.885, -408) -> (10.9983, -413) projected
  circle A0 centre (268, -105.5) radius 15 projected
  circle A1 centre (180, -105.5) radius 15 projected
  circle A2 centre (92, -105.5) radius 15 projected
  circle A3 centre (76.5, -121) radius 1.75 projected
  circle A4 centre (107.5, -90) radius 1.75 projected
  circle A5 centre (164.5, -121) radius 1.75 projected
  circle A6 centre (195.5, -90) radius 1.75 projected
  circle A7 centre (283.5, -121) radius 1.75 projected
  circle A8 centre (283.5, -90) radius 1.75 projected
  circle A9 centre (252.5, -90) radius 1.75 projected
  circle A10 centre (252.5, -121) radius 1.75 projected
  circle A11 centre (164.5, -90) radius 1.75 projected
  circle A12 centre (195.5, -121) radius 1.75 projected
  circle A13 centre (76.5, -90) radius 1.75 projected
  circle A14 centre (107.5, -121) radius 1.75 projected
  line L635 (375, -480) -> (375, 0) projected
  line L636 (375, 0) -> (-15, 0) projected
  line L637 (-15, 0) -> (-15, -480) projected
  line L638 (-15, -480) -> (375, -480) projected
  circle A15 centre (100, -25) radius 1.75 projected
  circle A16 centre (180, -7.5) radius 1.75 projected
  circle A17 centre (-7.5, -65) radius 1.75 projected
  circle A18 centre (-7.5, -415) radius 1.75 projected
  circle A19 centre (367.5, -65) radius 1.75 projected
  circle A20 centre (367.5, -415) radius 1.75 projected
  circle A21 centre (50, -7.5) radius 1.75 projected
  circle A22 centre (310, -7.5) radius 1.75 projected
  circle A23 centre (310, -472.5) radius 1.75 projected
  circle A24 centre (50, -472.5) radius 1.75 projected
  circle A25 centre (180, -25) radius 1.75 projected
  circle A26 centre (260, -25) radius 1.75 projected
  line L639 (2.25, -360) -> (2.25, -320) construction
  line L640 (0, -360) -> (0, -320)
  line L641 (4.5, -320) -> (4.5, -360)
  arc A27 (0, -360) -> (4.5, -360) centre (2.25, -360) ccw
  arc A28 (4.5, -320) -> (0, -320) centre (2.25, -320) ccw
  line L642 (12.5, -320) -> (12.5, -360)
  line L643 (10.25, -360) -> (10.25, -320) construction
  arc A29 (12.5, -320) -> (8, -320) centre (10.25, -320) ccw
  line L644 (8, -360) -> (8, -320)
  arc A30 (8, -360) -> (12.5, -360) centre (10.25, -360) ccw
  line L645 (20.5, -320) -> (20.5, -360)
  line L646 (18.25, -360) -> (18.25, -320) construction
  arc A31 (20.5, -320) -> (16, -320) centre (18.25, -320) ccw
  line L647 (16, -360) -> (16, -320)
  arc A32 (16, -360) -> (20.5, -360) centre (18.25, -360) ccw
  point P0 (0, 0)
  point P1 (2.25, -340)
  point P2 (10.25, -340)
  point P3 (18.25, -340)
  dimension "d75" = 4.5
  dimension "d76" = 120
  dimension "d77" = 40
  dimension "d78" = 15
  dimension "d81" = 8
  constraints: 24 end point, 12 point on circle, 6 centre point, 4 tangent, 1 horizontal, 1 midpoint, 1 parallel, 1 vertical, 24 other
  measures "d75" distance between parallel lines of L641 L640
  measures "d76" distance from line of L638 L639.start
  measures "d77" distance of L640.start L640.end
  measures "d78" distance between parallel lines of L637 L640
  measures "d81" distance of L641.start L642.start
extrude "Extrusion5" cut sketch "Sketch6" against normal through all contours L640 A28 L641 A27 | L642 A30 L644 A29 | L645 A32 L647 A31